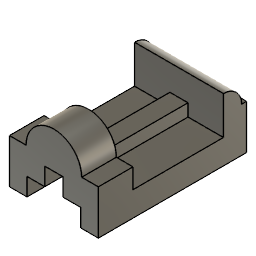
Design 2 Robocon Task 3 (Autodesk Fusion 360 design; units mm, degrees)
part number: 2026-03-05-20-50-21-525
Autodesk Fusion 360 part; units mm, degrees
sketch "Sketch1" plane through (0, 0, 0) normal (0, 0, 1) x (1, 0, 0)
  line L0 (-70, -60) -> (110, -60)
  line L1 (110, -60) -> (110, 240)
  line L2 (110, 240) -> (-70, 240)
  line L3 (-70, 240) -> (-70, -60)
  constraint horizontal L0
  constraint vertical L1
  constraint horizontal L2
  constraint vertical L3
extrude "Extrude1" add sketch "Sketch1" along normal blind 90
sketch "Sketch2" plane through (0, 0, 90) normal (0, 0, 1) x (-1, 0, 0)
  line L0 (70, -240) -> (70, 60)
  line L1 (70, 60) -> (-110, 60)
  line L2 (-110, 60) -> (-110, -240)
  line L3 (-110, -240) -> (70, -240)
  line L4 (70, -193.0373) -> (-110, -193.0373)
  line L5 (-110, -193.0373) -> (-110, -10.0813)
  line L6 (-110, -10.0813) -> (70, -10.0813)
  line L7 (70, -10.0813) -> (70, -193.0373)
  constraint horizontal L4
  constraint vertical L5
  constraint horizontal L6
  constraint vertical L7
  constraint coincident L2 L5.end
  constraint coincident L0 L4.start
extrude "Extrude2" cut sketch "Sketch2" against normal blind 40 contours L0 L2 L4 L5 L6 L7
sketch "Sketch3" plane through (0, 0, 0) normal (0, 1, 0) x (1, 0, 0)
sketch "Sketch4" plane through (0, -60, 0) normal (0, -1, 0) x (1, 0, 0)
  line L0 (-70, 0) -> (110, 0)
  line L1 (110, 0) -> (110, 90)
  line L2 (110, 90) -> (-70, 90)
  line L3 (-70, 90) -> (-70, 0)
  line L4 (-70, 0) -> (-34.3509, 0)
  line L5 (-34.3509, 0) -> (-34.3509, 36)
  line L6 (-34.3509, 36) -> (-18.3509, 36)
  line L7 (-70, 0) -> (110, 0)
  line L8 (-70, 0) -> (110, 0)
  line L9 (110, 0) -> (20, 0)
  line L10 (110, 0) -> (20, 0)
  line L11 (110, 0) -> (20, 0)
  line L12 (20, 0) -> (20, 23.3377)
  line L13 (110, 0) -> (74.3509, 0)
  line L14 (74.3509, 0) -> (74.3509, 36)
  line L15 (-18.3509, 36) -> (1.6491, 36)
  line L16 (1.6491, 36) -> (1.6491, 72)
  line L17 (58.3509, 36) -> (38.3509, 36)
  line L18 (74.3509, 36) -> (58.3509, 36)
  line L19 (38.3509, 36) -> (38.3509, 72)
  line L20 (1.6491, 72) -> (38.3509, 72)
  point P0 (20, 0)
  constraint coincident L0.start L3.end
  constraint coincident L0 L4.end
  constraint vertical L5
  constraint horizontal L6
  constraint coincident L0.end L1.start
  constraint midpoint L8 P0
  constraint coincident P0 L9.end
  constraint perpendicular L8 L12
  constraint symmetric L0.start L12 L0.end
  constraint symmetric L4.end L12 L13.end
  constraint perpendicular L15 L16
  constraint symmetric L5.end L12 L14.end
  constraint symmetric L6.end L12 L17.start
  constraint symmetric L12 L15.end L17.end
  constraint symmetric L12 L16.end L19.end
  constraint perpendicular L19 L20
extrude "Extrude3" cut sketch "Sketch4" against normal blind 400 contours L0 L5 L6 L7 L8 L9 L10 L11 L14 L15 L16 L17 L18 L19 L20
ref_plane "WorkPlane1" through (-70, -60, 90) normal (1, 0, 0) x (0, 1, 0)
sketch "Sketch5" plane through (-70, 0, 0) normal (1, 0, 0) x (0, 1, 0)
  arc A0 through (230, 90, 180) (219.1739, 116.1366, 180) (193.0373, 126.9627, 180)
  line L0 (193.0373, 90, 180) -> (240, 90, 180)
  line L1 (193.0373, 90, 180) -> (230, 90, 180) construction
  line L2 (193.0373, 90, 180) -> (193.0373, 126.9627, 180) construction
  line L3 (193.0373, 126.9627, 180) -> (193.0373, 90, 180)
  point P0 (193.0373, 90)
  dimension "d12" = 90
sketch "Sketch6" plane through (0, 240, 0) normal (0, 1, 0) x (-1, 0, 0)
  line L0 (34.3509, 36) -> (34.3509, 0)
  line L1 (34.3509, 0) -> (70, 0)
  line L2 (70, 0) -> (70, 90)
  line L3 (70, 90) -> (-110, 90)
  line L4 (-110, 90) -> (-110, 0)
  line L5 (-110, 0) -> (-74.3509, 0)
  line L6 (-74.3509, 0) -> (-74.3509, 36)
  line L7 (-74.3509, 36) -> (-38.3509, 36)
  line L8 (-38.3509, 36) -> (-38.3509, 72)
  line L9 (-38.3509, 72) -> (-1.6491, 72)
  line L10 (-1.6491, 72) -> (-1.6491, 36)
  line L11 (-1.6491, 36) -> (34.3509, 36)
extrude "Extrude4" add sketch "Sketch5" against normal blind 180 contours A0 L0 L3 in plane through (110, 0, 0) normal (1, 0, 0)
ref_plane "WorkPlane2" through (-70, 10.0813, 90) normal (0, 1, 0) x (-1, 0, 0)
sketch "Sketch7" plane through (0, 10.0813, 0) normal (0, 1, 0) x (1, 0, 0)
  line L0 (110, -90) -> (-70, -90)
  line L1 (-70, -90) -> (20, -90)
  arc A0 (-36.2753, -90) -> (76.2753, -90) centre (20, -90) ccw
  point P0 (-70, -90)
  constraint coincident P0 L0.end
  constraint midpoint L0 L1.end
  constraint coincident L0 A0.end
  constraint coincident L1 A0.start
  constraint coincident L1.end A0.centre
sketch "Sketch8" plane through (-70, 0, 0) normal (-1, 0, 0) x (0, -1, 0)
  line L0 (-10.0813, 90) -> (-10.0813, 50)
  line L1 (-10.0813, 50) -> (-193.0373, 50)
  line L2 (-193.0373, 50) -> (-193.0373, 126.9627)
  arc A0 (-193.0373, 126.9627) -> (-230, 90) centre (-193.0373, 90) ccw
  line L3 (-230, 90) -> (-240, 90)
  line L4 (-240, 90) -> (-240, 0)
  line L5 (-240, 0) -> (60, 0)
  line L6 (60, 0) -> (60, 90)
  line L7 (60, 90) -> (-10.0813, 90)
ref_plane "WorkPlane3" through (20, -24.9594, 45) normal (0, -1, 0) x (1, 0, 0)
extrude "Extrude5" add sketch "Sketch7" against normal blind 10
mirror "Mirror1" about plane through (20, -24.9594, 45) normal (0, -1, 0) of "Extrude5"
extrude "Extrude6" add 1 faces at (25.576, 0.0813, 126.9941) along direction (0, -1, 0) blind 54
ref_plane "WorkPlane4" through (110, 193.0373, 50) normal (0, 0, 1) x (1, 0, 0)
sketch "Sketch9" plane through (0, 0, 50) normal (0, 0, 1) x (1, 0, 0)
  line L0 (1.6491, 193.0373) -> (38.3509, 193.0373)
  line L1 (38.3509, 193.0373) -> (38.3509, 10.0813)
  line L2 (38.3509, 10.0813) -> (1.6491, 10.0813)
  line L3 (1.6491, 10.0813) -> (1.6491, 193.0373)
  point P0 (1.6491, 193.0373)
  point P1 (38.3509, 10.0813)
  constraint horizontal L0
  constraint vertical L1
  constraint horizontal L2
  constraint vertical L3
  constraint coincident P1 L1.end
  constraint coincident P0 L0.start
extrude "Extrude7" add sketch "Sketch9" along normal blind 25
